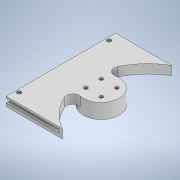
# Autodesk Inventor part: ECHO SOUNDER HOLDER FINAL DESIGN (revised)
Saved by Autodesk Inventor 2020.4 (Build 244396000, 396)
## iProperties
Created: 2021-06-17
Part Number: ECHO SOUNDER HOLDER FINAL DESIGN (revised)
Material: Generic
Document SubType Name: Modeling
Designer: Brandon
Density: 1 g/cm^3
Appearance: Default
Author: Brandon
Autodesk Inventor part; units mm, degrees
ref_plane "YZ Plane" through (0, 0, 0) normal (1, 0, 0) x (0, 1, 0)
ref_plane "XZ Plane" through (0, 0, 0) normal (0, 1, 0) x (-1, 0, 0)
ref_plane "XY Plane" through (0, 0, 0) normal (0, 0, 1) x (1, 0, 0)
sketch "Sketch1" plane through (0, 0, 0) normal (0, 1, 0) x (-1, 0, 0)
  arc A0 (52.6783, -85) -> (52.6783, 85) centre (0, 0) ccw
  circle A1 centre (130, 70) radius 3
  circle A2 centre (130, -70) radius 3
  line L0 (52.6783, 85) -> (135, 85)
  line L1 (52.6783, -85) -> (135, -85)
  line L2 (135, -85) -> (135, 85)
  circle A3 centre (72.25, 0) radius 25.25
  circle A4 centre (72.25, 0) radius 27.75
  arc A5 (47.7624, -85) -> (47.7624, 85) centre (0, 0) ccw
  line L3 (52.6783, 85) -> (47.7624, 85)
  line L4 (52.6783, -85) -> (47.7624, -85)
  point P0 (100, 0)
  point P1 (96.583, -13.3404)
  point P2 (96.583, 13.3404)
  dimension "d9" = 6
  dimension "d10" = 6
  dimension "d29" = 50.5
  dimension "d30" = 55.5
  constraints: 10 end point, 6 centre point, 4 point on circle, 3 coincident, 1 horizontal, 1 perpendicular, 1 point on line
  measures "d9" diameter of A1
  measures "d10" diameter of A2
  measures "d29" diameter of A3
  measures "d30" diameter of A4
extrude "Extrusion1" add sketch "Sketch1" along normal blind 3 contours A0 L0 L2 L1 | A3
extrude "Extrusion3" add sketch "Sketch1" along normal blind 3 and the other way blind 20 contours A4 A5 | A5 A4
extrude "Extrusion4" add sketch "Sketch1" along normal blind 3 and the other way blind 6 contours L4 A5 A4 A0 | A4 A5 L3 A0
sketch "Sketch3" plane through (0, -6, 0) normal (0, -1, 0) x (1, 0, 0)
  arc A0 (-96.583, -13.3404) -> (-47.7624, -85) centre (0, 0) ccw projected
  line L0 (0, 0) -> (-135, 0)
  line L1 (-135, -85) -> (-135, 85) projected
  line L2 (-135, 0) -> (-135, 85)
  line L3 (-135, 85) -> (-47.7624, 85) projected
  line L4 (-135, 85) -> (-47.7624, 85)
  line L5 (-47.7624, -85) -> (-135, -85) projected
  line L6 (-135, 0) -> (-135, -85)
  line L7 (-135, -85) -> (-47.7624, -85)
  arc A1 (-47.7624, 85) -> (-47.7624, -85) centre (0, 0) ccw
  circle A2 centre (-130, -70) radius 3 projected
  circle A3 centre (-130, -70) radius 3
  circle A4 centre (-130, 70) radius 3 projected
  circle A5 centre (-130, 70) radius 3
  point P0 (-96.583, -13.3404)
  dimension "d40" = 135
  constraints: 10 end point, 3 centre point, 2 coincident, 2 collinear, 2 point on circle, 1 midpoint, 1 perpendicular, 1 vertical
  measures "d40" distance of L0.start L0.end
extrude "Extrusion5" add sketch "Sketch3" along normal blind 5
sketch "Sketch6" plane through (-72.25, 0, 0) normal (0, -1, 0) x (1, 0, 0)
  circle A0 centre (0, 0) radius 25.25
  point P0 (72.25, 0)
  constraints: 1 centre point
extrude "Extrusion6" add sketch "Sketch6" along normal blind 2
sketch "Sketch7" plane through (0, 3, 0) normal (0, 1, 0) x (1, 0, 0)
  arc A0 (-96.583, -13.3404) -> (-96.583, 13.3404) centre (-72.25, 0) ccw projected
  line L0 (-72.25, 0) -> (-72.25, -12)
  line L1 (-72.25, -12) -> (-60.25, -12)
  line L2 (-60.25, -12) -> (-60.25, 12)
  line L3 (-60.25, 12) -> (-84.25, 12)
  line L4 (-84.25, 12) -> (-84.25, -12)
  point P0 (0, 0)
  dimension "d57" = 12
  dimension "d58" = 12
  dimension "d59" = 24
  dimension "d60" = 24
  dimension "d61" = 24
  constraints: 10 end point, 3 perpendicular, 1 point on line, 1 vertical
  measures "d57" distance of L0.start L0.end
  measures "d58" distance of L0.end L1.end
  measures "d59" distance of L1.end L2.end
  measures "d60" distance of L2.end L3.end
  measures "d61" distance of L3.end L4.end
hole "Hole2" at (-60.25, 3, 12) at (-60.25, 3, -12) at (-84.25, 3, -12) at (-84.25, 3, 12) direction (0, -1, 0) diameter 3.5 end through all counterbore diameter 5.5 counterbore depth 3
fillet "Fillet1" radius 10 2 edges at (-96.583, -4, -13.3404) (-96.583, -4, 13.3404)
body "Solid1"
